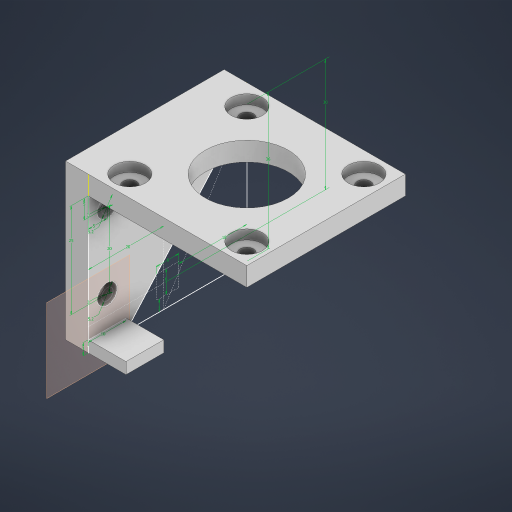
# Autodesk Inventor part: CoreXY Stepper Holder
Saved by Autodesk Inventor 2024.2 (Build 282272000, 272)
## iProperties
Created: 2024-10-03
Part Number: CoreXY Stepper Holder
Material: Generic
Document SubType Name: Modeling
Designer: jerem
Density: 1 g/cm^3
Appearance: Default
Author: jerem
Autodesk Inventor part; units mm, degrees
ref_plane "YZ Plane" through (0, 0, 0) normal (1, 0, 0) x (0, 1, 0)
ref_plane "XZ Plane" through (0, 0, 0) normal (0, 1, 0) x (-1, 0, 0)
ref_plane "XY Plane" through (0, 0, 0) normal (0, 0, 1) x (1, 0, 0)
sketch "Sketch1" plane through (0, 0, 0) normal (0, 1, 0) x (-1, 0, 0)
  line L0 (-21, -21) -> (21, -21)
  line L1 (21, -21) -> (21, 21)
  line L2 (21, 21) -> (-21, 21)
  line L3 (-21, 21) -> (-21, -21)
  line L4 (-21, -21) -> (21, 21) construction
  line L5 (21, -21) -> (-21, 21) construction
  circle A0 centre (15.5, 15.5) radius 1.75
  circle A1 centre (15.5, -15.5) radius 1.75
  circle A2 centre (-15.5, -15.5) radius 1.75
  circle A3 centre (-15.5, 15.5) radius 1.75
  circle A4 centre (0, 0) radius 11
  circle A5 centre (0, 0) radius 4 construction
  line L6 (21, -17) -> (17, -21)
  line L7 (21, 17) -> (17, 21)
  line L8 (-17, -21) -> (-21, -17)
  line L9 (-21, 17) -> (-17, 21)
  circle A6 centre (0, 0) radius 2.5 construction
  circle A7 centre (44, -10) radius 4 construction
  line L10 (44, -10) -> (44, 10) construction
  circle A8 centre (44, -10) radius 7.5 construction
  circle A9 centre (44, 10) radius 11.15 construction
  circle A10 centre (44, 10) radius 3.5 construction
  circle A11 centre (52, 10) radius 1.5 construction
  line L11 (52, 10) -> (44, 10) construction
  circle A12 centre (44, 18) radius 1.5 construction
  circle A13 centre (36, 10) radius 1.5 construction
  circle A14 centre (44, 2) radius 1.5 construction
  circle A15 centre (44, 10) radius 5.1 construction
  line L12 (44, 0) -> (21, 0) construction
  circle A16 centre (-15.5, -15.5) radius 4.15
  circle A17 centre (-15.5, 15.5) radius 4.15
  circle A18 centre (15.5, -15.5) radius 4.15
  circle A19 centre (15.5, 15.5) radius 4.15
  line L13 (21, -21) -> (24, -21)
  line L14 (21, 21) -> (21, -21)
  line L15 (27, -21) -> (27, 21)
  line L16 (24, -21) -> (27, -21)
  line L17 (21, 21) -> (27, 21)
  dimension "d0" = 42
  dimension "d1" = 31
  dimension "d2" = 31
  dimension "d3" = 31
  dimension "d4" = 31
  dimension "d5" = 3.5
  dimension "d6" = 3.5
  dimension "d7" = 3.5
  dimension "d8" = 3.5
  dimension "d9" = 22
  dimension "d10" = 8
  dimension "d11" = 4
  dimension "d12" = 4
  dimension "d13" = 4
  dimension "d14" = 4
  dimension "d15" = 4
  dimension "d16" = 4
  dimension "d17" = 4
  dimension "d18" = 5
  dimension "d21" = 8
  dimension "d23" = 20
  dimension "d24" = 15
  dimension "d28" = 22.3
  dimension "d29" = 7
  dimension "d30" = 3
  dimension "d31" = 8
  dimension "d32" = 360
  dimension "d33" = 10.2
  dimension "d36" = 2.4
  dimension "d38" = 2.4
  dimension "d39" = 2.4
  dimension "d40" = 2.4
  dimension "d46" = 17
  dimension "d47" = 6
  constraints: 36 end point, 20 centre point, 13 coincident, 11 point on line, 6 horizontal, 4 midpoint, 4 perpendicular, 2 parallel, 2 vertical, 9 other
  measures "d0" distance of L0.end L1.end
  measures "d1" distance of A1.centre A0.centre
  measures "d2" distance of A2.centre A1.centre
  measures "d3" distance of A3.centre A2.centre
  measures "d4" distance of A0.centre A3.centre
  measures "d5" diameter of A0
  measures "d6" diameter of A1
  measures "d7" diameter of A2
  measures "d8" diameter of A3
  measures "d9" diameter of A4
  measures "d10" diameter of A5
  measures "d11" distance of L0.end L6.end
  measures "d12" distance of L0.end L6.start
  measures "d13" distance of L1.end L7.end
  measures "d14" distance of L7.start L1.end
  measures "d15" distance of L3.start L9.end
  measures "d16" distance of L3.start L9.start
  measures "d17" distance of L3.end L8.end
  measures "d18" diameter of A6
  measures "d21" diameter of A7
  measures "d23" distance of L10.start L10.end
  measures "d24" diameter of A8
  measures "d28" diameter of A9
  measures "d29" diameter of A10
  measures "d30" diameter of A11
  measures "d31" distance of L11.start L11.end
  measures "d33" diameter of A15
  measures "d36" radial gap between concentric circles of A17 A3
  measures "d38" radial gap between concentric circles of A19 A0
  measures "d39" radial gap between concentric circles of A2 A16
  measures "d40" radial gap between concentric circles of A18 A1
  measures "d46" distance between parallel lines of L10 L15
  measures "d47" distance between parallel lines of L1 L15
extrude "Extrusion1" add sketch "Sketch1" along normal blind 5 contours L3 L8 L0 | L8 L3 L9 L2 L7 L1 L6 L0 | L6 L1 L0 | L3 L2 L9 | L1 L17 L15 L16 L13 | L7 L2 L1
extrude "Extrusion2" add sketch "Sketch1" along normal blind 2.5 contours A16 | A17 | A18 | A19
ref_plane "Work Plane1" through (-21, -30, 21) normal (1, 0, 0) x (0, 0, -1)
sketch "Sketch2" plane through (-21, -30, 21) normal (1, 0, 0) x (0, 0, -1)
  line L0 (42, 30) -> (42, -6)
  line L1 (20, 30) -> (20, -6) construction
  circle A0 centre (5, 25) radius 2.6
  circle A1 centre (5, 25) radius 1.5
  circle A2 centre (5, 5) radius 2.6
  circle A3 centre (5, 5) radius 1.5
  line L2 (0, 30) -> (0, 35) projected
  line L3 (0, 30) -> (42, 30) projected
  line L4 (0, 30) -> (42, 30)
  line L5 (42, 30) -> (42, -6)
  line L6 (42, -6) -> (0, -6)
  line L7 (0, -6) -> (0, 30)
  line L8 (42, 30) -> (42, 35) projected
  line L9 (42, 30) -> (20, -6) construction
  line L10 (20, 0) -> (0, 0) construction
  line L11 (0, -6) -> (10, -6)
  line L12 (10, -6) -> (10, -3)
  line L13 (10, -3) -> (0, -3)
  line L14 (0, -3) -> (0, -6)
  line L15 (18, 3) -> (24, 3) construction
  line L16 (24, 3) -> (24, -3) construction
  line L17 (24, -3) -> (18, -3) construction
  line L18 (18, -3) -> (18, 3) construction
  line L19 (42, 30) -> (10, -6)
  point P0 (21, 30)
  point P1 (0, -4.5)
  point P2 (0, -3)
  point P3 (10, -6)
  point P4 (10, -6)
  dimension "d51" = 5.2
  dimension "d52" = 3
  dimension "d59" = 5.2
  dimension "d60" = 3
  dimension "d64" = 5
  dimension "d66" = 5
  dimension "d67" = 20
  dimension "d68" = 25
  dimension "d69" = 20
  dimension "d70" = 36
  dimension "d71" = 30
  dimension "d72" = 10
  dimension "d73" = 3
  dimension "d76" = 18
  dimension "d77" = 6
  dimension "d78" = 6
  dimension "d79" = 3
  constraints: 32 end point, 6 parallel, 4 centre point, 4 perpendicular, 4 point on line, 3 horizontal, 2 coincident, 1 collinear, 1 midpoint
  measures "d51" diameter of A0
  measures "d52" diameter of A1
  measures "d59" diameter of A2
  measures "d60" diameter of A3
  measures "d64" distance from line of L2 A1.centre
  measures "d66" distance from line of L3 A0.centre
  measures "d67" distance of A0.centre A2.centre
  measures "d68" vertical distance of L2.start A2.centre
  measures "d69" distance between parallel lines of L7 L1
  measures "d70" distance between parallel lines of L3 L6
  measures "d71" distance between parallel lines of L3 L10
  measures "d72" distance from line of point (0, -4.5) L12
  measures "d73" distance between parallel lines of L11 L13
  measures "d76" distance between parallel lines of L0 L16
  measures "d77" distance between parallel lines of L17 L15
  measures "d78" distance between parallel lines of L16 L18
  measures "d79" distance between parallel lines of L6 L17
extrude "Extrusion4" add sketch "Sketch2" against normal up to surface (6 mm away) contours L19 L12 L13 L7 L3 | L6 L7 L13 L12
extrude "Extrusion5" add sketch "Sketch2" along normal blind 3 from surface at -6 contours A0 | A2
extrude "Extrusion6" add sketch "Sketch2" along normal blind 10 contours L6 L7 L13 L12
equation "\"d2\" = d1"
equation "\"d3\" = d1"
equation "\"d4\" = d1"
equation "\"d6\" = d5"
equation "\"d7\" = d5"
equation "\"d8\" = d5"
equation "\"d12\" = d11"
equation "\"d13\" = d11"
equation "\"d14\" = d11"
equation "\"d15\" = d11"
equation "\"d16\" = d11"
equation "\"d17\" = d11"
body "Solid1"
